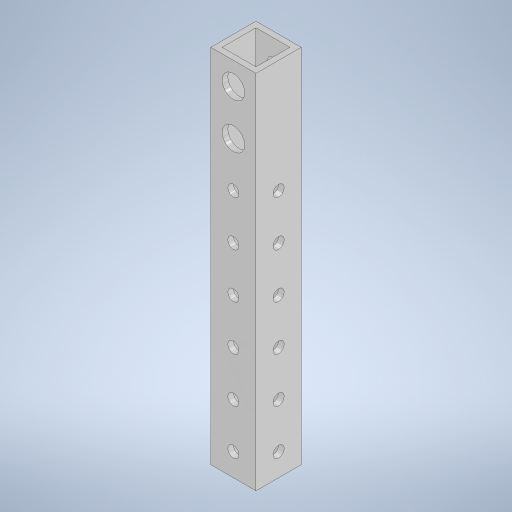
# Autodesk Inventor part: testRoboRescue_Chassis_Frame_heightBar
Saved by Autodesk Inventor 2023 (Build 270158000, 158)
## iProperties
Created: 2022-03-14
Part Number: testRoboRescue_Chassis_Frame_heightBar
Material: Aluminum 6061
Document SubType Name: Modeling
Designer: Nebil Oumer
Density: 2.7 g/cm^3
Appearance: Aluminum - Polished
Mass: 199.103 g
Surface Area: 476.612 cm^2
Volume: 73.7418 cm^3
Author: Nebil Oumer
Autodesk Inventor part; units mm, degrees
ref_plane "YZ Plane" through (0, 0, 0) normal (1, 0, 0) x (0, 1, 0)
ref_plane "XZ Plane" through (0, 0, 0) normal (0, 1, 0) x (-1, 0, 0)
ref_plane "XY Plane" through (0, 0, 0) normal (0, 0, 1) x (1, 0, 0)
sketch "Sketch2" plane through (0, 0, 0) normal (0, 0, 1) x (1, 0, 0)
  line L0 (0, 0) -> (25.4, 0)
  line L1 (25.4, 0) -> (25.4, 25.4)
  line L2 (25.4, 25.4) -> (0, 25.4)
  line L3 (0, 25.4) -> (0, 0)
  line L4 (3.175, 22.225) -> (22.225, 22.225)
  line L5 (22.225, 22.225) -> (22.225, 3.175)
  line L6 (22.225, 3.175) -> (3.175, 3.175)
  line L7 (3.175, 3.175) -> (3.175, 22.225)
  dimension "d0" = 25.4
  dimension "d1" = 25.4
  dimension "d2" = 3.175
  constraints: 16 end point, 4 parallel, 2 perpendicular, 1 horizontal, 3 other
  measures "d0" distance of L2.end L1.end
  measures "d1" distance of L0.end L1.end
  measures "d2" distance between parallel lines of L2 L4
extrude "Extrusion1" add sketch "Sketch2" along normal blind 203.2
sketch "Sketch5" plane through (0, 0, 0) normal (-1, 0, 0) x (0, 0, 1)
  circle A0 centre (139.7, 12.7) radius 3.175
  line L0 (203.2, 25.4) -> (203.2, 0) projected
  line L1 (0, 25.4) -> (203.2, 25.4) projected
  circle A1 centre (114.3, 12.7) radius 3.175
  circle A2 centre (88.9, 12.7) radius 3.175
  circle A3 centre (63.5, 12.7) radius 3.175
  circle A4 centre (38.1, 12.7) radius 3.175
  circle A5 centre (12.7, 12.7) radius 3.175
  point P0 (0, 0)
  point P1 (203.2, 12.7)
  point P2 (203.2, 12.7)
  dimension "d13" = 6.35
  dimension "d15" = 63.5
  dimension "d23" = 25.4
  constraints: 6 centre point, 2 midpoint, 1 horizontal, 1 horizontal alignment, 10 other
  measures "d13" diameter of A0
  measures "d15" distance from line of L0 A0.centre
  measures "d23" distance of A0.centre A1.centre
extrude "Extrusion4" cut sketch "Sketch5" against normal through all
sketch "Sketch6" plane through (0, 25.4, 0) normal (0, 1, 0) x (1, 0, 0)
  line L0 (25.4, -203.2) -> (0, -203.2) projected
  line L1 (0, 0) -> (0, -203.2) projected
  point P0 (12.7, -190.5)
  dimension "d28" = 12.7
  dimension "d29" = 12.7
  measures "d28" distance from line of L0 point (12.7, -190.5)
  measures "d29" distance from line of L1 point (12.7, -190.5)
hole "Hole1" at (12.7, 25.4, 190.5) direction (0, -1, 0) diameter 6.35 end through all counterbore diameter 12.7 counterbore depth 6.35
pattern_linear "Rectangular Pattern1" count 2 spacing 25.4 along (0, 0, -1) of "Hole1"
sketch "Sketch7" plane through (0, 25.4, 0) normal (0, 1, 0) x (1, 0, 0)
  line L0 (25.4, -203.2) -> (0, -203.2) projected
  line L1 (0, 0) -> (0, -203.2) projected
  point P0 (12.7021, -139.7)
  dimension "d40" = 63.5
  dimension "d41" = 12.7021
  measures "d40" distance from line of L0 point (12.702, -139.7)
  measures "d41" distance from line of L1 point (12.702, -139.7)
hole "Hole2" at (12.7021, 25.4, 139.7) direction (0, -1, 0) diameter 6.35 end through all
pattern_linear "Rectangular Pattern2" count 6 spacing 25.4 along (0, 0, -1) of "Hole2"
equation "\"d0\" = d1"
body "Solid1"
